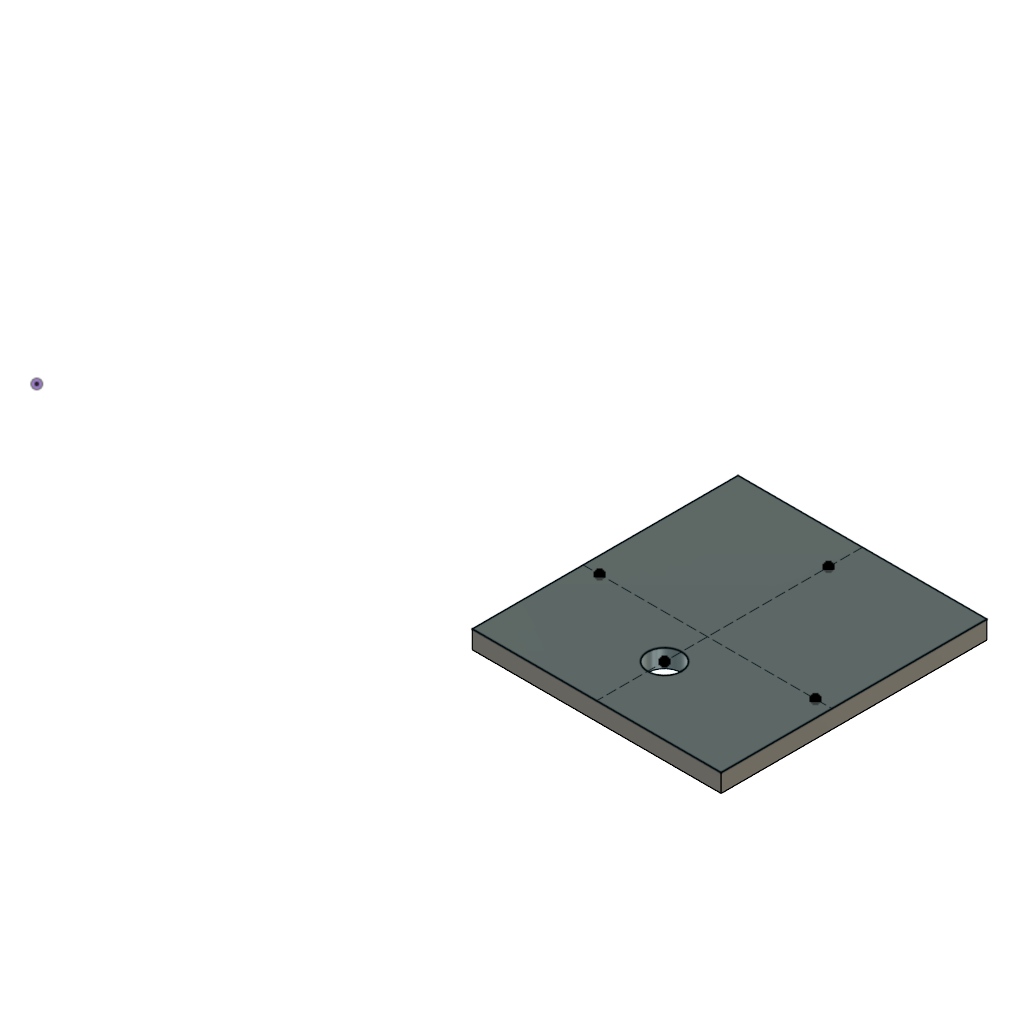
Adapter (Autodesk Fusion 360 design; units mm, degrees)
Autodesk Fusion 360 part; units mm, degrees
sketch "Skizze1" plane through (0, 0, 0) normal (0, 0, 1) x (1, 0, 0)
  line L0 (38, 23.99) -> (60, 23.99)
  line L1 (60, 23.99) -> (60, 0.49)
  line L2 (60, 0.49) -> (38, 0.49)
  line L3 (38, 0.49) -> (38, 23.99)
  circle A0 centre (49, 6.49) radius 1.5
  line L4 (49, 23.99) -> (49, 0.49) construction
  line L5 (38, 10.29) -> (60, 10.29) construction
  point P0 (39.46, 10.29)
  point P1 (58.54, 10.29)
  point P2 (49, 20.99)
  dimension "d1" = 38
  dimension "d2" = 60
  dimension "d3" = 0.49
  dimension "d4" = 23.99
  dimension "d5" = 3
  dimension "d7" = 6.49
  dimension "d8" = 10.29
  dimension "d9" = 39.46
  dimension "d10" = 58.54
  dimension "d11" = 20.99
  constraint horizontal L0
  constraint vertical L1
  constraint horizontal L2
  constraint vertical L3
  constraint midpoint L0 L4.start
  constraint midpoint L2 L4.end
  constraint coincident L3 L5.start
  constraint coincident L1 L5.end
  constraint perpendicular L1 L5
  constraint coincident A0.centre L4
  constraint coincident L5 P0
  constraint coincident L5 P1
  constraint coincident L4 P2
  measures "d1" horizontal distance of origin L2.end
  measures "d2" horizontal distance of origin L1.end
  measures "d3" vertical distance of origin L2.end
  measures "d4" vertical distance of origin L0.start
  measures "d5" diameter of A0
  measures "d7" vertical distance of origin A0.centre
  measures "d8" vertical distance of origin L5.start
  measures "d9" horizontal distance of origin P0
  measures "d10" horizontal distance of origin P1
  measures "d11" vertical distance of origin P2
extrude "Extrusion1" add sketch "Skizze1" against normal blind 1.6
